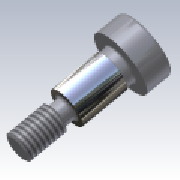
# Autodesk Inventor part: SCREW,SHOULDER,M8X8MM
Saved by Autodesk Inventor 2022.4 (Build 264492000, 492)
## iProperties
Company: Cooper Bussmann Denmark
Category: _
Manager: 611-42576
Created: 2001-02-28
Part Number: SCREW,SHOULDER,M8X8MM
Document SubType Name: Modeling
Designer: Peter Damgaard
Material: Steel, High Strength Low Alloy
Density: 7.84 g/cm^3
Appearance: Grey (Dark)
Mass: 10.7925 g
Surface Area: 9.51114 cm^2
Volume: 1.3766 cm^3
Mfg Approved By: Cathy.Lesperance
Engr Approved By: P
Checked By: 0002109114
User Status: Released
Description: SCREW,SHOULDER,M8X8MM
Control State: 0
Master: False
Checked Out: False
Shininess: 60.0
CN_MASS: 0.010793
FIRST_DESCRIPTION: SHOULDER DIAMETER 8MM, HEAD DIAMETER 13MM
SECOND_DESCRIPTION: THREAD M6 X1 X 11MM LG,  HEAD HEIGHT 6MM
THIRD_DESCRIPTION: WV
CN_SERVICEABLE: _
PTC_WM_ITERATION: 1
PTC_WM_ORGANIZATION_ID: CLWC
PTC_WM_LIFECYCLE: CLWC_CAD_LC
CL_runCount: 1
FinishProperty: ToBeSet
Density: 7.84
Volumn: 1.0724371659246204
Area: 8.535162991116971
PropertySet Name: Model Information
Author: -
Subject: 92981A198
Keywords: MCMASTER.CARR
Revision Number: A
Autodesk Inventor part; units mm, degrees
ref_plane "YZ Plane" through (0, 0, 0) normal (1, 0, 0) x (0, 1, 0)
ref_plane "XZ Plane" through (0, 0, 0) normal (0, 1, 0) x (-1, 0, 0)
ref_plane "XY Plane" through (0, 0, 0) normal (0, 0, 1) x (1, 0, 0)
sketch "Sketch1" plane through (0, 0, 0) normal (0, 0, 1) x (1, 0, 0)
  line L0 (0, 0) -> (-4, 0)
  line L1 (-4, 0) -> (-4, -6.15)
  line L2 (-4, -6.15) -> (0, -6.15)
  line L3 (0, -6.15) -> (0, 0)
  line L4 (0, 0) -> (-13.1356, 0) construction
  dimension "d1" = 6.15
  dimension "d2" = 4
  constraints: 10 end point, 2 parallel, 1 horizontal, 1 perpendicular, 1 point on line
  measures "d1" distance of L0.end L1.end
  measures "d2" distance of L0.start L0.end
revolve "Shoulder" add sketch "Sketch1" angle 360 about axis through (0, -6.15, 0) along (0, 1, 0)
sketch "Sketch2" plane through (0, 0, 0) normal (0, 1, 0) x (1, 0, 0)
  circle A0 centre (0, 0) radius 4 projected
  circle A1 centre (0, 0) radius 3.76
  dimension "d3" = 7.52
  constraints: 1 centre point, 1 concentric
  measures "d3" diameter of A1
extrude "Shoulder_neck" add sketch "Sketch2" along normal blind 1.85 contours A1
sketch "Sketch3" plane through (0, 1.85, 0) normal (0, 1, 0) x (1, 0, 0)
  circle A0 centre (0, 0) radius 3.76 projected
  circle A1 centre (0, 0) radius 6.6
  dimension "d6" = 13.2
  constraints: 1 centre point, 1 concentric
  measures "d6" diameter of A1
extrude "Head" add sketch "Sketch3" along normal blind 5.5 contours A0 | A1
sketch "Sketch4" plane through (0, -6.15, 0) normal (0, -1, 0) x (1, 0, 0)
  circle A0 centre (0, 0) radius 4 projected
  circle A1 centre (0, 0) radius 2.255
  dimension "d9" = 4.51
  constraints: 1 centre point, 1 concentric
  measures "d9" diameter of A1
extrude "Thread_neck" add sketch "Sketch4" along normal blind 2.3 contours A1
sketch "Sketch5" plane through (0, -8.45, 0) normal (0, -1, 0) x (1, 0, 0)
  circle A0 centre (0, 0) radius 2.255 projected
  circle A1 centre (0, 0) radius 3
  dimension "d12" = 6
  constraints: 1 centre point, 1 concentric
  measures "d12" diameter of A1
extrude "Thread_shoulder" add sketch "Sketch5" along normal blind 8.7 contours A0 | A1
sketch "Sketch6" plane through (0, 7.35, 0) normal (0, 1, 0) x (1, 0, 0)
  circle A0 centre (0, 0) radius 6.6 projected
  circle A1 centre (0, 0) radius 2 construction
  line L0 (-2, 1.1547) -> (-2, -1.1547)
  line L1 (-2, -1.1547) -> (0, -2.3094)
  line L2 (0, -2.3094) -> (2, -1.1547)
  line L3 (2, -1.1547) -> (2, 1.1547)
  line L4 (2, 1.1547) -> (0, 2.3094)
  line L5 (0, 2.3094) -> (-2, 1.1547)
  dimension "d15" = 4
  constraints: 12 end point, 6 equal length, 6 tangent, 1 centre point, 1 concentric, 1 parallel, 1 vertical
  measures "d15" diameter of A1
extrude "Hex" cut sketch "Sketch6" against normal blind 3.3 contours L5 L4 L3 L2 L1 L0
chamfer "Chamfer1" distance 0.24 angle 30 1 edges at (4, 0, 0) measured on face at (-3.8813, 0, -0.3191)
fillet "Fillet1" radius 0.4 1 edges at (-3.76, 1.85, 0)
chamfer "Chamfer2" distance 0.4 angle 30 1 edges at (-6.6, 7.35, 0) measured on face at (6.5145, 5.5167, 1.0587)
chamfer "Chamfer3" distance 0.5 angle 30 1 edges at (-3, -17.15, 0) measured on face at (-0.5351, -17.15, 1.0949)
fillet "Fillet2" radius 0.6 1 edges at (-2.255, -6.15, 0)
chamfer "Chamfer7" distance 0.745 angle 30 1 edges at (-3, -8.45, 0) measured on face at (2.7226, -8.45, -0.2393)
thread "Thread" size "M6x1" class "6g" standard "ANSI Metric M Profile" full length
equation "\"d3\" = Shoulder_neck_dia"
equation "\"d4\" = Shoulder_neck_length"
equation "\"d6\" = Head_diameter"
equation "\"d7\" = Head_height"
equation "\"d9\" = Thread_neck_dia"
equation "\"d10\" = Thread_neck_length"
equation "\"d12\" = Thread_diameter"
equation "\"d13\" = Thread_length - Thread_neck_length"
equation "\"d15\" = Hex_size"
equation "\"d16\" = Hex_length"
equation "\"d18\" = -0.5 * Shoulder_neck_dia + 0.5 * Shoulder_diameter"
equation "\"d64\" = -0.5 * Shoulder_neck_dia + 0.5 * Shoulder_diameter"
equation "\"d21\" = 0.1 * Hex_size"
equation "\"d65\" = 0.1 * Hex_size"
equation "\"d23\" = 0.5 * Thread_pitch"
equation "\"d66\" = 0.5 * Thread_pitch"
equation "\"d25\" = Thread_neck_radius"
equation "\"d60\" = -0.5 * Thread_neck_dia + 0.5 * Thread_diameter"
equation "\"d67\" = -0.5 * Thread_neck_dia + 0.5 * Thread_diameter"
equation "\"d1\" = Shoulder_length - Shoulder_neck_length"
equation "\"d2\" = 0.5 * Shoulder_diameter"
equation "\"Shoulder_diameter\" = 8"
equation "\"Shoulder_length\" = 8"
equation "\"Shoulder_neck_dia\" = 7.52"
equation "\"Thread_diameter\" = 6"
equation "\"Thread_length\" = 11"
equation "\"Head_diameter\" = 13.2"
equation "\"Head_height\" = 5.5"
equation "\"Thread_neck_dia\" = 4.51"
equation "\"Hex_size\" = 4"
equation "\"Hex_length\" = 3.3"
equation "\"Thread_pitch\" = 1"
equation "\"Shoulder_neck_length\" = 1.85"
equation "\"Thread_neck_length\" = 2.3"
equation "\"Thread_neck_radius\" = 0.6"
body "Solid1"
